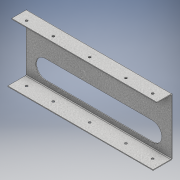
# Autodesk Inventor part: SidePanelCoverSpacer
Saved by Autodesk Inventor 2017 (Build 210142000, 142)
## iProperties
Created: 2017-10-09
Part Number: SidePanelCoverSpacer
Material: Generic
Document SubType Name: Modeling
Designer: Kathryn Rosie
Density: 1 g/cm^3
Appearance: Flat - Polished Gray
Author: Kathryn Rosie
Autodesk Inventor part; units mm, degrees
ref_plane "YZ Plane" through (0, 0, 0) normal (1, 0, 0) x (0, 1, 0)
ref_plane "XZ Plane" through (0, 0, 0) normal (0, 1, 0) x (-1, 0, 0)
ref_plane "XY Plane" through (0, 0, 0) normal (0, 0, 1) x (1, 0, 0)
sketch "Sketch1" plane through (0, 0, 0) normal (1, 0, 0) x (0, 1, 0)
  line L0 (10, 150) -> (48, 150)
  line L1 (50, 148) -> (50, 2)
  line L2 (48, 0) -> (0, 0)
  line L3 (0, 2) -> (46, 2)
  line L4 (48, 4) -> (48, 146)
  line L5 (46, 148) -> (10, 148)
  line L6 (0, 0) -> (0, 2)
  line L7 (10, 150) -> (10, 148)
  arc A0 (48, 146) -> (46, 148) centre (46, 146) ccw
  arc A1 (50, 148) -> (48, 150) centre (48, 148) ccw
  arc A2 (48, 0) -> (50, 2) centre (48, 2) ccw
  arc A3 (46, 2) -> (48, 4) centre (46, 4) ccw
  point P0 (50, 150)
  point P1 (50, 0)
  dimension "d0" = 40
  dimension "d1" = 150
  dimension "d2" = 50
  dimension "d3" = 2
  dimension "d4" = 2
  constraints: 16 end point, 8 point on circle, 8 tangent, 4 centre point, 4 perpendicular, 4 point on line, 3 equal radius, 1 coincident, 1 horizontal, 1 parallel, 1 vertical, 2 other
  measures "d0" distance of L0.start point (50, 150)
  measures "d1" distance of point (50, 150) point (50, 0)
  measures "d2" distance of point (50, 0) L2.end
  measures "d3" distance between parallel lines of L1 L4
  measures "d4" radius of A0
extrude "Extrusion1" add sketch "Sketch1" along normal blind 380
sketch "Sketch2" plane through (0, 50, 148) normal (0, 1, 0) x (1, 0, 0)
  line L0 (330, 108) -> (50, 108) construction
  line L1 (330, 83) -> (50, 83)
  line L2 (50, 133) -> (330, 133)
  arc A0 (330, 83) -> (330, 133) centre (330, 108) ccw
  arc A1 (50, 133) -> (50, 83) centre (50, 108) ccw
  line L3 (0, 146) -> (380, 146) projected
  line L4 (0, 144) -> (0, 2) projected
  line L5 (380, 146) -> (380, 0) projected
  line L6 (0, 148) -> (380, 148) projected
  point P0 (190, 108)
  dimension "d7" = 280
  dimension "d8" = 190
  dimension "d9" = 50
  dimension "d10" = 40
  constraints: 8 end point, 4 point on circle, 4 tangent, 2 centre point, 1 horizontal, 1 midpoint, 1 parallel
  measures "d7" distance of L0.end L0.start
  measures "d8" distance from line of L5 point (190, 108)
  measures "d9" distance between parallel lines of L2 L1
  measures "d10" distance from line of L6 point (190, 108)
extrude "Extrusion2" cut sketch "Sketch2" against normal up to surface (2 mm away)
sketch "Sketch3" plane through (0, 0, 0) normal (0, 0, -1) x (-1, 0, 0)
  line L0 (0, 0) -> (-380, 0) projected
  line L1 (-380, 0) -> (-380, 48) projected
  point P0 (-355, 24)
  point P1 (-285, 24)
  point P2 (-190, 24)
  point P3 (-25, 24)
  point P4 (-95, 24)
  dimension "d13" = 24
  dimension "d14" = 70
  dimension "d15" = 95
  dimension "d16" = 95
  dimension "d17" = 70
  dimension "d18" = 25
  constraints: 4 horizontal alignment
  measures "d13" distance from line of L0 point (-355, 24)
  measures "d14" distance of point (-285, 24) point (-355, 24)
  measures "d15" distance of point (-190, 24) point (-285, 24)
  measures "d16" distance of point (-95, 24) point (-190, 24)
  measures "d17" distance of point (-25, 24) point (-95, 24)
  measures "d18" distance from line of L1 point (-355, 24)
hole "Hole1" at (355, 24, 0) at (285, 24, 0) at (190, 24, 0) at (25, 24, 0) at (95, 24, 0) direction (0, 0, 1) diameter 6 end through all
body "Solid1"
